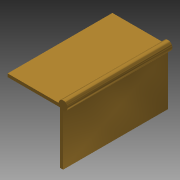
# Autodesk Inventor part: Hinge_Rear
Saved by Autodesk Inventor 2013 (Build 170138000, 138)
## iProperties
Created: 2015-07-03
Part Number: Hinge_Rear
Material: Brass, Soft Yellow
Document SubType Name: Modeling
Designer: Kyle
Density: 8.47 g/cm^3
Mass: 4.87754 g
Surface Area: 14.8733 cm^2
Volume: 0.57586 cm^3
Author: Kyle
Autodesk Inventor part; units mm, degrees
ref_plane "YZ Plane" through (0, 0, 0) normal (1, 0, 0) x (0, 1, 0)
ref_plane "XZ Plane" through (0, 0, 0) normal (0, 1, 0) x (-1, 0, 0)
ref_plane "XY Plane" through (0, 0, 0) normal (0, 0, 1) x (1, 0, 0)
sketch "Sketch1" plane through (0, 0, 0) normal (0, 0, 1) x (1, 0, 0)
  line L0 (0, 0) -> (12.7, 0)
  line L1 (12.7, 0) -> (12.7, -12.7)
  line L2 (0, 0.762) -> (12.3844, 0.762)
  line L3 (13.462, -0.3156) -> (13.462, -12.7)
  line L4 (0, 0.762) -> (0, 0)
  line L5 (12.7, -12.7) -> (13.462, -12.7)
  arc A0 (13.462, -0.3156) -> (12.3844, 0.762) centre (13.462, 0.762) ccw
  dimension "d0" = 12.7
  dimension "d1" = 12.7
  dimension "d2" = 0.762
  constraints: 12 end point, 3 perpendicular, 2 point on circle, 1 centre point, 1 horizontal, 1 parallel
  measures "d0" distance of L0.start L0.end
  measures "d1" distance of L0.end L1.end
  measures "d2" distance between parallel lines of L2 L0
extrude "Extrusion1" add sketch "Sketch1" along normal blind 25.4
body "Solid1"
